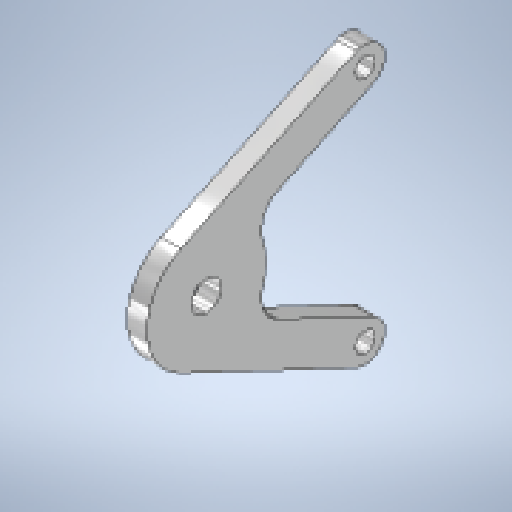
# Autodesk Inventor part: Frame (Motor Side)
Saved by Autodesk Inventor 2023.1 (Build 271208000, 208)
## iProperties
Created: 2022-05-22
Part Number: Frame (Motor Side)
Material: Aluminum 6061
Document SubType Name: Modeling
Designer: Nathan Cai
Density: 2.7 g/cm^3
Appearance: Aluminum - Flat
Mass: 43.7998 g
Surface Area: 76.8958 cm^2
Volume: 16.2221 cm^3
C2C: 2.250 in
Author: Nathan Cai
Autodesk Inventor part; units mm, degrees
ref_plane "YZ Plane" through (0, 0, 0) normal (1, 0, 0) x (0, 1, 0)
ref_plane "XZ Plane" through (0, 0, 0) normal (0, 1, 0) x (-1, 0, 0)
ref_plane "XY Plane" through (0, 0, 0) normal (0, 0, 1) x (1, 0, 0)
sketch "Sketch1" plane through (0, 0, 0) normal (1, 0, 0) x (0, 1, 0)
  circle A0 centre (0, 0) radius 4.7625 construction
  line L0 (0, 0) -> (0, 57.15) construction
  circle A1 centre (0, 57.15) radius 4.7625
  circle A2 centre (0, 57.15) radius 76.2 construction
  circle A3 centre (0, 57.15) radius 19.05
  line L1 (0, 6.35) -> (38.1, 6.35) construction
  circle A4 centre (38.1, 6.35) radius 3.175
  circle A5 centre (38.1, 6.35) radius 6.35
  line L2 (17.2181, 65.3011) -> (43.8394, 9.067)
  line L3 (13.4243, 43.6337) -> (32.3606, 3.633)
  circle A6 centre (-38.1, 6.35) radius 3.175
  circle A7 centre (-38.1, 6.35) radius 6.35
  line L4 (-17.2181, 65.3011) -> (-43.8394, 9.067)
  line L5 (-13.4243, 43.6337) -> (-32.3606, 3.633)
  line L6 (38.1, 12.7) -> (-38.1, 12.7) construction
  line L7 (-38.1, 0) -> (38.1, 0) construction
  line L8 (38.1, 6.35) -> (17.5542, 49.7504) construction
  point P0 (44.2067, 4.609)
  point P1 (-17.0485, 35.9779)
  point P2 (-17.2181, 65.3011)
  point P3 (-13.4243, 43.6337)
  point P4 (28.0683, 12.7)
  point P5 (-28.0683, 12.7)
  dimension "d0" = 9.525
  dimension "C2C" = 57.15
  dimension "d3" = 9.525
  dimension "d4" = 152.4
  dimension "d5" = 38.1
  dimension "d6" = 38.1
  dimension "d7" = 6.35
  dimension "d8" = 12.7
  dimension "d9" = 6.35
  dimension "d10" = 12.7
  constraints: 18 end point, 12 point on circle, 8 centre point, 8 coincident, 7 symmetric about line, 6 tangent, 2 parallel, 2 point on line, 1 horizontal, 1 vertical, 2 other
  measures "d0" diameter of A0
  measures "C2C" distance of L0.start L0.end
  measures "d3" diameter of A1
  measures "d4" diameter of A2
  measures "d5" diameter of A3
  measures "d6" distance of L1.start L1.end
  measures "d7" diameter of A4
  measures "d8" diameter of A5
  measures "d9" distance from line of A0.centre L1
  measures "d10" distance between parallel lines of L2 L3
extrude "Extrusion1" add sketch "Sketch1" along normal blind 6.35
fillet "Fillet1" radius 9.525 2 edges at (3.175, 13.4243, 43.6337) (3.175, -13.4243, 43.6337)
equation "\"d10\" = d8"
body "Solid1"
